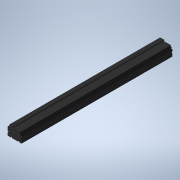
# Autodesk Inventor part: EGC-80-TB85678GK0--0---0_0_R0L22000
Saved by Autodesk Inventor 2021 (Build 250183000, 183)
## iProperties
Created: 2026-04-25
Part Number: EGC-80-TB85678GK0--0---0_0_R0L22000
Material: Generic
Catalog Web Link: www.3dfindit.com
Description: EGC_R-EGC rohr
Vendor: FESTO
Document SubType Name: Modeling
Designer: psAdmin
Manufacturer: FESTO
Mass: 3404.6 g
Surface Area: 3458.7 cm^2
Volume: 3404.6 cm^3
Density: 1 g/cm^3
Appearance: PSOLRGB-176-176-176
Category: PARTsolutions
Company: FESTO
Title: EGC-80-TB85678GK0--0--0_0_R
Author: Cadenas PARTsolutions
Comments: EGC rohr
PSOL_IDENT_0: {$CADENAS_DATA/23d-libs/festo/parts/e/egc/parts/egc_fa_rohr.prj},364 {VTYP=3D},{NB=EGC-80-TB85678GK0
PSOL_IDENT_1: --0---0_0_R0L22000},{LINA=EGC-80-TB85678GK0--0--0_0_R},{NN=EGC_R},{DATE=13.04.2021 11:17:45},{GEOMDA
PSOL_IDENT_2: TE=13.04.2021 11:17:00},{VERSION=},{LINEID=30},{WBVAR=FKT,L,L2,SL,HR,ZSL,ZSR,FSA,K,AM,SA,WMS,ZUBA,ZU
PSOL_IDENT_3: BC,HGO,HGOK,HGOANMO,HGOANZBEF,HGOANZHWRP,EHMYM,HGOYL11},{WBNUMERIC=L,L2,HR,K,ZUBA,ZUBC,HGO,HGOK,HGOA
PSOL_IDENT_4: NZBEF,HGOANZHWRP,EHMYM,HGOYL11}  {NB=EGC-80-TB85678GK0--0---0_0_R0L22000},{LINA=EGC-80-TB85678GK0--0
PSOL_IDENT_5: --0_0_R},{KT=DUMMY},{HEAD=EGC},{BG=80},{VER=3.000},{FKT=TB},{L=856},{LM=[50:10000]},{L2=78},{L6=2.00
PSOL_IDENT_6: 0},{L10=120},{LSF=70.000},{L1SF=90.000},{LHWS=135.000},{LZUBA=70.000},{LZUBC=45.000},{SL=GK},{TYPSL=
PSOL_IDENT_7: 120},{HR=0},{ZSL=-},{ZSR=-},{FSA=-},{L11=0},{K=0},{AM=},{SA=-},{WMS=-},{ZUBA=0},{ZUBC=0},{HGO=0},{HG
PSOL_IDENT_8: OL3=65.000},{HGOK=0},{HGOK1=173.000},{HGOK2=147.000},{HGOK3=151.000},{HGOBWB1=50.000},{HGOHWB1=40.00
PSOL_IDENT_9: 0},{HGOE=0},{HGOUEHMYRP=612},{HGOANMO=L},{HGOANZBEF=2},{HGOANZHWRP=2},{EHMYM=0},{HGOYL11=0},{HGODIST
PSOL_IDENT_10: MIT=153},{BSL7=17.000},{HGOBLECHL=-11.500},{HGODISTMP=15},{ERDUNG=213},{WMS1='-','M1','M2'}
NB: EGC-80-TB85678GK0--0---0_0_R0L22000
NN: EGC_R
NT: EGC rohr
NBSYN: $HEAD.-$BG.-$FKT.$L.$L2.$SL.$HR.$ZSL.$ZSR.$K.$FSA.$AM.$SA.$WMS.$ZUBA._$ZUBC._R$HGO.$HGOANMO.$HGOANZBEF.$HGOANZHWRP.$HGOK.$EHMYM.$HGOYL11.
LINA: EGC-80-TB85678GK0--0--0_0_R
CATALOG: Festo
HEAD: EGC
BG: 80
FKT: TB
L: 856
L2: 78
L6: 2
LSF: 70
L1SF: 90
LHWS: 135
LZUBA: 70
LZUBC: 45
SL: GK
HR: 0
ZSL: -
ZSR: -
FSA: -
K: 0
SA: -
WMS: -
ZUBA: 0
ZUBC: 0
HGO: 0
HGOL3: 65
HGOK: 0
HGOK1: 173
HGOK2: 147
HGOK3: 151
HGOBWB1: 50
HGOHWB1: 40
HGOE: 0
HGOANMO: L
HGOANZBEF: 2
HGOANZHWRP: 2
EHMYM: 0
HGOYL11: 0
BSL7: 17
HGOBLECHL: -11.5
SUPPLIER: FESTO
ARTICLENO: EGC-80-TB85678GK0--0---0_0_R0L22000
BOMINFO: EGC-80-TB85678GK0--0--0_0_R
CREATOR: CADENAS GmbH
Autodesk Inventor part; units mm, degrees
sketch "Sketch_1" plane through (0, 0, 0) normal (0, 0, 1) x (1, 0, 0)
  line L0 (0, 45.4) -> (0, 0)
  line L1 (0, 0) -> (80, 0)
  line L2 (80, 0) -> (80, 35.5)
  line L3 (80, 35.5) -> (72.0728, 52.5)
  line L4 (72.0728, 52.5) -> (34, 52.5)
  line L5 (34, 52.5) -> (34, 60)
  line L6 (34, 60) -> (10, 60)
  line L7 (10, 60) -> (10, 52.5)
  line L8 (10, 52.5) -> (9.2, 52.5)
  line L9 (9.2, 52.5) -> (9.2, 52.9)
  line L10 (9.2, 52.9) -> (8.0011, 52.9)
  line L11 (8.0011, 52.9) -> (6.5, 50.3)
  line L12 (6.5, 50.3) -> (6.5, 45.4)
  line L13 (6.5, 45.4) -> (0, 45.4)
  constraints: 28 end point
extrude "Extrusion1" add sketch "Sketch_1" against normal blind 856
sketch "Sketch_2" plane through (0, 0, 0) normal (0, 0, 1) x (1, 0, 0)
  line L0 (-5, 65) -> (-5, -5)
  line L1 (-5, -5) -> (85, -5)
  line L2 (85, -5) -> (85, 65)
  line L3 (85, 65) -> (-5, 65)
  arc A0 (0, 1) -> (1, 0) centre (1, 1) ccw
  line L4 (1, 0) -> (17, 0)
  arc A1 (17, 0) -> (17.5, 0.5) centre (17, 0.5) ccw
  line L5 (17.5, 0.5) -> (17.5, 1.3)
  arc A2 (17.5, 1.3) -> (17, 1.8) centre (17, 1.3) ccw
  line L6 (17, 1.8) -> (14.95, 1.8)
  arc A3 (14.4197, 3.0803) -> (14.95, 1.8) centre (14.95, 2.55) ccw
  line L7 (14.4197, 3.0803) -> (16.8607, 5.5213)
  arc A4 (18.982, 6.4) -> (16.8607, 5.5213) centre (18.982, 3.4) ccw
  line L8 (18.982, 6.4) -> (21.018, 6.4)
  arc A5 (23.1393, 5.5213) -> (21.018, 6.4) centre (21.018, 3.4) ccw
  line L9 (23.1393, 5.5213) -> (25.5803, 3.0803)
  arc A6 (25.05, 1.8) -> (25.5803, 3.0803) centre (25.05, 2.55) ccw
  line L10 (25.05, 1.8) -> (23, 1.8)
  arc A7 (23, 1.8) -> (22.5, 1.3) centre (23, 1.3) ccw
  line L11 (22.5, 1.3) -> (22.5, 0.5)
  arc A8 (22.5, 0.5) -> (23, 0) centre (23, 0.5) ccw
  line L12 (23, 0) -> (57, 0)
  arc A9 (57, 0) -> (57.5, 0.5) centre (57, 0.5) ccw
  line L13 (57.5, 0.5) -> (57.5, 1.3)
  arc A10 (57.5, 1.3) -> (57, 1.8) centre (57, 1.3) ccw
  line L14 (57, 1.8) -> (54.95, 1.8)
  arc A11 (54.4197, 3.0803) -> (54.95, 1.8) centre (54.95, 2.55) ccw
  line L15 (54.4197, 3.0803) -> (56.8607, 5.5213)
  arc A12 (58.982, 6.4) -> (56.8607, 5.5213) centre (58.982, 3.4) ccw
  line L16 (58.982, 6.4) -> (61.018, 6.4)
  arc A13 (63.1393, 5.5213) -> (61.018, 6.4) centre (61.018, 3.4) ccw
  line L17 (63.1393, 5.5213) -> (65.5803, 3.0803)
  arc A14 (65.05, 1.8) -> (65.5803, 3.0803) centre (65.05, 2.55) ccw
  line L18 (65.05, 1.8) -> (63, 1.8)
  arc A15 (63, 1.8) -> (62.5, 1.3) centre (63, 1.3) ccw
  line L19 (62.5, 1.3) -> (62.5, 0.5)
  arc A16 (62.5, 0.5) -> (63, 0) centre (63, 0.5) ccw
  line L20 (63, 0) -> (79, 0)
  arc A17 (79, 0) -> (80, 1) centre (79, 1) ccw
  line L21 (80, 1) -> (80, 17)
  arc A18 (80, 17) -> (79.5, 17.5) centre (79.5, 17) ccw
  line L22 (79.5, 17.5) -> (78.7, 17.5)
  arc A19 (78.7, 17.5) -> (78.2, 17) centre (78.7, 17) ccw
  line L23 (78.2, 17) -> (78.2, 14.95)
  arc A20 (76.9197, 14.4197) -> (78.2, 14.95) centre (77.45, 14.95) ccw
  line L24 (76.9197, 14.4197) -> (74.4787, 16.8607)
  arc A21 (73.6, 18.982) -> (74.4787, 16.8607) centre (76.6, 18.982) ccw
  line L25 (73.6, 18.982) -> (73.6, 21.018)
  arc A22 (74.4787, 23.1393) -> (73.6, 21.018) centre (76.6, 21.018) ccw
  line L26 (74.4787, 23.1393) -> (76.9197, 25.5803)
  arc A23 (78.2, 25.05) -> (76.9197, 25.5803) centre (77.45, 25.05) ccw
  line L27 (78.2, 25.05) -> (78.2, 23)
  arc A24 (78.2, 23) -> (78.7, 22.5) centre (78.7, 23) ccw
  line L28 (78.7, 22.5) -> (79.5, 22.5)
  arc A25 (79.5, 22.5) -> (80, 23) centre (79.5, 23) ccw
  line L29 (80, 23) -> (80, 35.1009)
  arc A26 (80, 35.1009) -> (79.8314, 35.8617) centre (78.2, 35.1009) ccw
  line L30 (79.8314, 35.8617) -> (78.8589, 37.947)
  arc A27 (78.8589, 37.947) -> (78.3274, 38.1405) centre (78.4964, 37.778) ccw
  line L31 (78.3274, 38.1405) -> (77.6929, 37.8447)
  arc A28 (77.6929, 37.8447) -> (77.5962, 37.5789) centre (77.7775, 37.6634) ccw
  line L32 (77.5962, 37.5789) -> (77.9993, 36.7144)
  arc A29 (77.8997, 36.1495) -> (77.9993, 36.7144) centre (77.5462, 36.5031) ccw
  line L33 (77.8997, 36.1495) -> (75.4481, 33.6979)
  arc A30 (73.3268, 35.8192) -> (75.4481, 33.6979) centre (74.3875, 34.7586) ccw
  line L34 (73.3268, 35.8192) -> (74.2663, 36.7588)
  arc A31 (74.2663, 36.7588) -> (74.3161, 37.0412) centre (74.0896, 36.9355) ccw
  line L35 (74.3161, 37.0412) -> (72.3082, 41.3471)
  arc A32 (72.5017, 41.8787) -> (72.3082, 41.3471) centre (72.6708, 41.5162) ccw
  line L36 (72.5017, 41.8787) -> (74.8581, 42.9775)
  arc A33 (75.1239, 42.8808) -> (74.8581, 42.9775) centre (74.9426, 42.7963) ccw
  line L37 (75.1239, 42.8808) -> (75.2295, 42.6542)
  arc A34 (75.2295, 42.6542) -> (75.4953, 42.5575) centre (75.4108, 42.7387) ccw
  line L38 (75.4953, 42.5575) -> (76.1297, 42.8533)
  arc A35 (76.1297, 42.8533) -> (76.3232, 43.3849) centre (75.9607, 43.2158) ccw
  line L39 (76.3232, 43.3849) -> (75.3089, 45.56)
  arc A36 (75.3089, 45.56) -> (74.7774, 45.7535) centre (74.9464, 45.391) ccw
  line L40 (74.7774, 45.7535) -> (74.143, 45.4577)
  arc A37 (74.143, 45.4577) -> (74.0462, 45.1919) centre (74.2275, 45.2764) ccw
  line L41 (74.0462, 45.1919) -> (74.1519, 44.9653)
  arc A38 (74.0551, 44.6995) -> (74.1519, 44.9653) centre (73.9706, 44.8808) ccw
  line L42 (74.0551, 44.6995) -> (71.6987, 43.6007)
  arc A39 (71.1672, 43.7942) -> (71.6987, 43.6007) centre (71.5297, 43.9632) ccw
  line L43 (71.1672, 43.7942) -> (68.7582, 48.9601)
  arc A40 (68.9517, 49.4917) -> (68.7582, 48.9601) centre (69.1208, 49.1292) ccw
  line L44 (68.9517, 49.4917) -> (71.3081, 50.5905)
  arc A41 (71.5739, 50.4938) -> (71.3081, 50.5905) centre (71.3926, 50.4093) ccw
  line L45 (71.5739, 50.4938) -> (71.6796, 50.2672)
  arc A42 (71.6796, 50.2672) -> (71.9453, 50.1705) centre (71.8608, 50.3517) ccw
  line L46 (71.9453, 50.1705) -> (72.5798, 50.4663)
  arc A43 (72.5798, 50.4663) -> (72.7732, 50.9979) centre (72.4107, 50.8288) ccw
  line L47 (72.7732, 50.9979) -> (72.342, 51.9226)
  arc A44 (72.342, 51.9226) -> (71.4357, 52.5) centre (71.4357, 51.5) ccw
  line L48 (71.4357, 52.5) -> (32.597, 52.5)
  line L49 (32.597, 52.5) -> (32.3776, 52.88)
  line L50 (32.3776, 52.88) -> (33.4831, 57.0055)
  arc A45 (34, 58.664) -> (33.4831, 57.0055) centre (34.27, 57.67) ccw
  line L51 (34, 58.664) -> (34, 59.4)
  line L52 (34, 59.4) -> (31.4814, 59.4)
  arc A46 (29.936, 60) -> (31.4814, 59.4) centre (30.93, 60.27) ccw
  line L53 (29.936, 60) -> (14.064, 60)
  arc A47 (12.5186, 59.4) -> (14.064, 60) centre (13.07, 60.27) ccw
  line L54 (12.5186, 59.4) -> (10, 59.4)
  line L55 (10, 59.4) -> (10, 58.664)
  arc A48 (10.5169, 57.0055) -> (10, 58.664) centre (9.73, 57.67) ccw
  line L56 (10.5169, 57.0055) -> (11.6224, 52.88)
  line L57 (11.6224, 52.88) -> (10, 50.07)
  line L58 (10, 50.07) -> (10, 49.5)
  line L59 (10, 49.5) -> (11.3, 49.5)
  line L60 (11.3, 49.5) -> (11.3, 49.4)
  line L61 (11.3, 49.4) -> (11, 49.4)
  arc A49 (11, 49.4) -> (10.5, 48.9) centre (11, 48.9) ccw
  line L62 (10.5, 48.9) -> (10.5, 47.9)
  arc A50 (10, 47.4) -> (10.5, 47.9) centre (10, 47.9) ccw
  line L63 (10, 47.4) -> (9.8, 47.4)
  arc A51 (9.3, 47.9) -> (9.8, 47.4) centre (9.8, 47.9) ccw
  line L64 (9.3, 47.9) -> (9.3, 48.4046)
  arc A52 (9.3, 48.4046) -> (9.0692, 48.8259) centre (8.8, 48.4046) ccw
  arc A53 (8.9577, 50.0882) -> (9.0692, 48.8259) centre (9.5, 49.5) ccw
  arc A54 (8.9577, 50.0882) -> (9.1112, 50.369) centre (8.6188, 50.4558) ccw
  line L65 (9.1112, 50.369) -> (9.4954, 52.5479)
  arc A55 (9.4954, 52.5479) -> (9.2, 52.9) centre (9.2, 52.6) ccw
  line L66 (9.2, 52.9) -> (8.2898, 52.9)
  arc A56 (8.2898, 52.9) -> (7.8568, 52.65) centre (8.2898, 52.4) ccw
  line L67 (7.8568, 52.65) -> (6.567, 50.416)
  arc A57 (6.567, 50.416) -> (6.5, 50.166) centre (7, 50.166) ccw
  line L68 (6.5, 50.166) -> (6.5, 45.4)
  line L69 (6.5, 45.4) -> (1, 45.4)
  arc A58 (1, 45.4) -> (0, 44.4) centre (1, 44.4) ccw
  line L70 (0, 44.4) -> (0, 23)
  arc A59 (0, 23) -> (0.5, 22.5) centre (0.5, 23) ccw
  line L71 (0.5, 22.5) -> (1.3, 22.5)
  arc A60 (1.3, 22.5) -> (1.8, 23) centre (1.3, 23) ccw
  line L72 (1.8, 23) -> (1.8, 25.05)
  arc A61 (3.0803, 25.5803) -> (1.8, 25.05) centre (2.55, 25.05) ccw
  line L73 (3.0803, 25.5803) -> (5.5213, 23.1393)
  arc A62 (6.4, 21.018) -> (5.5213, 23.1393) centre (3.4, 21.018) ccw
  line L74 (6.4, 21.018) -> (6.4, 18.982)
  arc A63 (5.5213, 16.8607) -> (6.4, 18.982) centre (3.4, 18.982) ccw
  line L75 (5.5213, 16.8607) -> (3.0803, 14.4197)
  arc A64 (1.8, 14.95) -> (3.0803, 14.4197) centre (2.55, 14.95) ccw
  line L76 (1.8, 14.95) -> (1.8, 17)
  arc A65 (1.8, 17) -> (1.3, 17.5) centre (1.3, 17) ccw
  line L77 (1.3, 17.5) -> (0.5, 17.5)
  arc A66 (0.5, 17.5) -> (0, 17) centre (0.5, 17) ccw
  line L78 (0, 17) -> (0, 1)
  constraints: 158 end point, 134 point on circle, 67 centre point
extrude "Extrusion2" cut sketch "Sketch_2" against normal blind 856
sketch "Sketch_7" plane through (0, 0, 0) normal (0, 0, 1) x (1, 0, 0)
  line L0 (5.5, 45.4) -> (5.5, 44.4)
  line L1 (5.5, 44.4) -> (7.5, 44.4)
  line L2 (7.5, 44.4) -> (7.5, 46.4)
  line L3 (7.5, 46.4) -> (6.5, 46.4)
  arc A0 (5.5, 45.4) -> (6.5, 46.4) centre (5.5, 46.4) ccw
  constraints: 8 end point, 2 point on circle, 1 centre point
extrude "Extrusion3" add sketch "Sketch_7" against normal blind 856
ref_plane "ABP_XY" through (120, 20, 0) normal (0, 0, 1) x (1, 0, 0)
ref_plane "ABP_YZ" through (120, 20, 0) normal (1, 0, 0) x (0, 1, 0)
ref_plane "ABP_ZX" through (120, 20, 0) normal (0, 1, 0) x (0, 0, 1)
ref_plane "ABP_S1_XY" through (116.2523, 52.4047, 0) normal (0, 0, 1) x (0.4226, -0.9063, 0)
ref_plane "ABP_S1_YZ" through (116.2523, 52.4047, 0) normal (0.4226, -0.9063, 0) x (0.9063, 0.4226, 0)
ref_plane "ABP_S1_ZX" through (116.2523, 52.4047, 0) normal (0.9063, 0.4226, 0) x (0, 0, 1)
ref_plane "CLIP_XY" through (110.2934, 65.1837, -20) normal (0, 0, 1) x (0.9063, 0.4226, 0)
ref_plane "CLIP_YZ" through (110.2934, 65.1837, -20) normal (0.9063, 0.4226, 0) x (-0.4226, 0.9063, 0)
ref_plane "CLIP_ZX" through (110.2934, 65.1837, -20) normal (-0.4226, 0.9063, 0) x (0, 0, 1)
ref_plane "DISTANZSTUECK_XY" through (20.2, 59, -856) normal (0, 0, -1) x (1, 0, 0)
ref_plane "DISTANZSTUECK_YZ" through (20.2, 59, -856) normal (1, 0, 0) x (0, -1, 0)
ref_plane "DISTANZSTUECK_ZX" through (20.2, 59, -856) normal (0, -1, 0) x (0, 0, -1)
ref_plane "K_BINDER_XY" through (80, 20, -108) normal (-1, 0, 0) x (0, 0, -1)
ref_plane "K_BINDER_YZ" through (80, 20, -108) normal (0, 0, -1) x (0, -1, 0)
ref_plane "K_BINDER_ZX" through (80, 20, -108) normal (0, -1, 0) x (-1, 0, 0)
ref_plane "K_BINDER1_XY" through (80, 20, -258) normal (-1, 0, 0) x (0, 0, -1)
ref_plane "K_BINDER1_YZ" through (80, 20, -258) normal (0, 0, -1) x (0, -1, 0)
ref_plane "K_BINDER1_ZX" through (80, 20, -258) normal (0, -1, 0) x (-1, 0, 0)
ref_plane "MASS_XY" through (0, 42.4, -428) normal (1, 0, 0) x (0, 0, -1)
ref_plane "MASS_YZ" through (0, 42.4, -428) normal (0, 0, -1) x (0, 1, 0)
ref_plane "MASS_ZX" through (0, 42.4, -428) normal (0, 1, 0) x (1, 0, 0)
ref_plane "NST_XY" through (160, 20, -20) normal (-1, 0, 0) x (0, 0, -1)
ref_plane "NST_YZ" through (160, 20, -20) normal (0, 0, -1) x (0, -1, 0)
ref_plane "NST_ZX" through (160, 20, -20) normal (0, -1, 0) x (-1, 0, 0)
ref_plane "PB_XY" through (86, 12, -428) normal (0, 1, 0) x (1, 0, 0)
ref_plane "PB_YZ" through (86, 12, -428) normal (1, 0, 0) x (0, 0, -1)
ref_plane "PB_ZX" through (86, 12, -428) normal (0, 0, -1) x (0, 1, 0)
ref_plane "SD_HALTER_L_XY" through (22, 60, 0) normal (0, 0, 1) x (1, 0, 0)
ref_plane "SD_HALTER_L_YZ" through (22, 60, 0) normal (1, 0, 0) x (0, 1, 0)
ref_plane "SD_HALTER_L_ZX" through (22, 60, 0) normal (0, 1, 0) x (0, 0, 1)
ref_plane "SD_HALTER_R_XY" through (22, 60, -856) normal (0, 0, -1) x (1, 0, 0)
ref_plane "SD_HALTER_R_YZ" through (22, 60, -856) normal (1, 0, 0) x (0, -1, 0)
ref_plane "SD_HALTER_R_ZX" through (22, 60, -856) normal (0, -1, 0) x (0, 0, -1)
ref_plane "SENSORHALTER_L_XY" through (80, 20, -100.5) normal (-1, 0, 0) x (0, 0, -1)
ref_plane "SENSORHALTER_L_YZ" through (80, 20, -100.5) normal (0, 0, -1) x (0, -1, 0)
ref_plane "SENSORHALTER_L_ZX" through (80, 20, -100.5) normal (0, -1, 0) x (-1, 0, 0)
ref_plane "SENSORHALTER_R_XY" through (80, 20, -755.5) normal (-1, 0, 0) x (0, 0, -1)
ref_plane "SENSORHALTER_R_YZ" through (80, 20, -755.5) normal (0, 0, -1) x (0, -1, 0)
ref_plane "SENSORHALTER_R_ZX" through (80, 20, -755.5) normal (0, -1, 0) x (-1, 0, 0)
ref_plane "SENSOR_L_XY" through (69.9627, 46.3772, -43) normal (0, 0, 1) x (0.9063, 0.4226, 0)
ref_plane "SENSOR_L_YZ" through (69.9627, 46.3772, -43) normal (0.9063, 0.4226, 0) x (-0.4226, 0.9063, 0)
ref_plane "SENSOR_L_ZX" through (69.9627, 46.3772, -43) normal (-0.4226, 0.9063, 0) x (0, 0, 1)
ref_plane "SENSOR_R_XY" through (73.5127, 38.7642, -813) normal (0, 0, -1) x (0.9063, 0.4226, 0)
ref_plane "SENSOR_R_YZ" through (73.5127, 38.7642, -813) normal (0.9063, 0.4226, 0) x (0.4226, -0.9063, 0)
ref_plane "SENSOR_R_ZX" through (73.5127, 38.7642, -813) normal (0.4226, -0.9063, 0) x (0, 0, -1)
ref_plane "STECKDOSE_XY" through (160, 0, 0) normal (0, 0, 1) x (1, 0, 0)
ref_plane "STECKDOSE_YZ" through (160, 0, 0) normal (1, 0, 0) x (0, 1, 0)
ref_plane "STECKDOSE_ZX" through (160, 0, 0) normal (0, 1, 0) x (0, 0, 1)
ref_plane "TO_DUMMY_XY" through (40, 0, -428) normal (0, -1, 0) x (1, 0, 0)
ref_plane "TO_DUMMY_YZ" through (40, 0, -428) normal (1, 0, 0) x (0, 0, 1)
ref_plane "TO_DUMMY_ZX" through (40, 0, -428) normal (0, 0, 1) x (0, -1, 0)
ref_plane "TO_SLIDE_XY" through (22, 53, -778) normal (0, 0, 1) x (1, 0, 0)
ref_plane "TO_SLIDE_YZ" through (22, 53, -778) normal (1, 0, 0) x (0, 1, 0)
ref_plane "TO_SLIDE_ZX" through (22, 53, -778) normal (0, 1, 0) x (0, 0, 1)
ref_plane "TO_SLIDE_EXPT_XY" through (22, 53, -794) normal (0, 0, 1) x (1, 0, 0)
ref_plane "TO_SLIDE_EXPT_YZ" through (22, 53, -794) normal (1, 0, 0) x (0, 1, 0)
ref_plane "TO_SLIDE_EXPT_ZX" through (22, 53, -794) normal (0, 1, 0) x (0, 0, 1)
ref_plane "TO_SLIDE_L_XY" through (22, 53, -658) normal (0, 0, 1) x (1, 0, 0)
ref_plane "TO_SLIDE_L_YZ" through (22, 53, -658) normal (1, 0, 0) x (0, 1, 0)
ref_plane "TO_SLIDE_L_ZX" through (22, 53, -658) normal (0, 1, 0) x (0, 0, 1)
ref_plane "TO_SLIDE_R_XY" through (22, 53, -898) normal (0, 0, 1) x (1, 0, 0)
ref_plane "TO_SLIDE_R_YZ" through (22, 53, -898) normal (1, 0, 0) x (0, 1, 0)
ref_plane "TO_SLIDE_R_ZX" through (22, 53, -898) normal (0, 1, 0) x (0, 0, 1)
ref_plane "ZR1_XY" through (40, 0, 0) normal (0, 0, 1) x (1, 0, 0)
ref_plane "ZR1_YZ" through (40, 0, 0) normal (1, 0, 0) x (0, 1, 0)
ref_plane "ZR1_ZX" through (40, 0, 0) normal (0, 1, 0) x (0, 0, 1)
ref_plane "ZR2_XY" through (40, 0, -856) normal (0, 0, -1) x (1, 0, 0)
ref_plane "ZR2_YZ" through (40, 0, -856) normal (1, 0, 0) x (0, -1, 0)
ref_plane "ZR2_ZX" through (40, 0, -856) normal (0, -1, 0) x (0, 0, -1)
body "Solid1"
